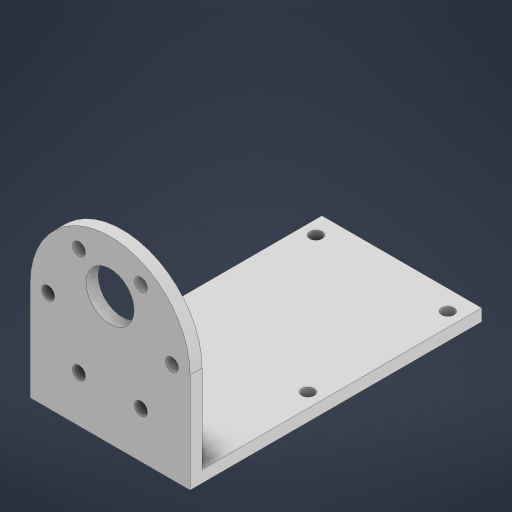
# Autodesk Inventor part: Push_motor_fix
Saved by Autodesk Inventor 2023 (Build 270158000, 158)
## iProperties
Created: 2023-11-09
Part Number: Push_motor_fix
Material: Generic
Document SubType Name: Modeling
Designer: Abhinav
Density: 1 g/cm^3
Appearance: Default
Author: Abhinav
Autodesk Inventor part; units mm, degrees
ref_plane "YZ Plane" through (0, 0, 0) normal (1, 0, 0) x (0, 1, 0)
ref_plane "XZ Plane" through (0, 0, 0) normal (0, 1, 0) x (-1, 0, 0)
ref_plane "XY Plane" through (0, 0, 0) normal (0, 0, 1) x (1, 0, 0)
sketch "Sketch1" plane through (0, 0, 0) normal (0, 0, 1) x (1, 0, 0)
  circle A0 centre (15.5, -7) radius 1.6
  circle A1 centre (7.75, -20.4234) radius 1.6
  circle A2 centre (-7.75, -20.4234) radius 1.6
  circle A3 centre (-15.5, -7) radius 1.6
  circle A4 centre (7.75, 6.4234) radius 1.6
  circle A5 centre (-7.75, 6.4234) radius 1.6
  circle A6 centre (0, 0) radius 6
  arc A7 (20, -7) -> (-20, -7) centre (0, -7) ccw
  line L0 (20, -7) -> (20, -32)
  line L1 (20, -32) -> (-20, -32)
  line L2 (-20, -32) -> (-20, -7)
  dimension "d0" = 40
  dimension "d1" = 25
  constraints: 8 centre point, 6 end point, 2 point on circle, 1 parallel
  measures "d0" diameter of A7
  measures "d1" distance of L0.start L0.end
extrude "Extrusion1" add sketch "Sketch1" along normal blind 3
sketch "Sketch2" plane through (-20, -32, 0) normal (0, -1, 0) x (1, 0, 0)
  line L0 (0, 0) -> (0, 3) projected
  line L1 (0, 3) -> (40, 3)
  line L2 (40, 3) -> (40, -70)
  line L3 (40, -70) -> (0, -70)
  line L4 (0, -70) -> (0, 3)
  line L5 (0, -70) -> (40, -70)
  line L6 (40, -70) -> (40, -25)
  line L7 (40, -25) -> (0, -25) construction
  line L8 (0, -25) -> (0, -70)
  line L9 (40, -25) -> (0, -70) construction
  line L10 (36.5, -30) -> (3.5, -30) construction
  line L11 (3.5, -30) -> (3.5, -65) construction
  line L12 (3.5, -65) -> (36.5, -65) construction
  line L13 (36.5, -65) -> (36.5, -30) construction
  line L14 (36.5, -30) -> (3.5, -65) construction
  line L15 (3.5, -30) -> (36.5, -65) construction
  circle A0 centre (36.5, -30) radius 1.55
  circle A1 centre (36.5, -65) radius 1.55
  circle A2 centre (3.5, -30) radius 1.55
  circle A3 centre (3.5, -65) radius 1.55
  point P0 (20, 0)
  point P1 (20, -47.5)
  dimension "d4" = 73
  dimension "d5" = 45
  dimension "d6" = 33
  dimension "d7" = 35
  dimension "d8" = 3.1
  dimension "d11" = 35
  dimension "d14" = 33
  constraints: 30 end point, 6 parallel, 4 centre point, 4 horizontal, 3 midpoint, 3 perpendicular, 1 coincident, 1 point on line, 1 vertical, 6 other
  measures "d4" distance of L1.end L2.end
  measures "d5" distance of L6.end L5.end
  measures "d6" distance of L12.end L11.end
  measures "d7" distance of L11.end L10.end
  measures "d8" diameter of A0
  measures "d11" distance of A0.centre A1.centre
  measures "d14" distance of A0.centre A2.centre
extrude "Extrusion2" add sketch "Sketch2" against normal blind 3
body "Solid1"
